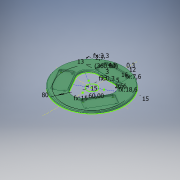
# Autodesk Inventor part: Stewart-Plate-inside
Saved by Autodesk Inventor 2018.2 (Build 222227000, 227)
## iProperties
Created: 2018-02-18
Part Number: Stewart-Plate-inside
Material: Generisch
Document SubType Name: Modeling
Designer: JochenAlt
Density: 1 g/cm^3
Appearance: Vorgabe
Author: JochenAlt
Autodesk Inventor part; units mm, degrees
ref_plane "YZ Plane" through (0, 0, 0) normal (1, 0, 0) x (0, 1, 0)
ref_plane "XZ Plane" through (0, 0, 0) normal (0, 1, 0) x (-1, 0, 0)
ref_plane "XY Plane" through (0, 0, 0) normal (0, 0, 1) x (1, 0, 0)
sketch "Skizze1" plane through (0, 0, 0) normal (0, 0, 1) x (1, 0, 0)
  line L0 (-56, 0) -> (56, 0) construction
  circle A0 centre (0, 0) radius 40
  line L1 (-8, 36) -> (8, 36)
  line L2 (8, 36) -> (8, 33)
  line L3 (8, 33) -> (-8, 33)
  line L4 (-8, 33) -> (-8, 36)
  line L5 (1.5, 33) -> (-1.5, 33)
  line L6 (-1.5, 33) -> (-1.5, 28)
  line L7 (-1.5, 28) -> (1.5, 28)
  line L8 (1.5, 28) -> (1.5, 33)
  circle A1 centre (0, 0) radius 7.5
  dimension "d9" = 80
  dimension "d10" = 3
  dimension "d11" = 33
  dimension "d14" = 16
  dimension "d23" = 5
  dimension "d62" = 15
  constraints: 16 end point, 4 parallel, 3 perpendicular, 2 centre point, 2 horizontal, 1 coincident, 1 midpoint, 1 point on line
  measures "d9" diameter of A0
  measures "d10" distance between parallel lines of L3 L1
  measures "d11" distance from line of L3 A0.centre
  measures "d14" distance between parallel lines of L2 L4
  measures "d23" distance between parallel lines of L3 L7
  measures "d62" diameter of A1
extrude "Extrusion3" add sketch "Skizze1" against normal blind 7 contours L1 L2 L3 L4 | L3 L8 L7 L6
fillet "Rundung1" radius 4 2 edges at (-8, 34.5, -7) (8, 34.5, -7)
sketch "Skizze2" plane through (-8, 36, 0) normal (0, 1, 0) x (1, 0, 0)
  circle A0 centre (3, 4) radius 1.1
  circle A1 centre (13, 4) radius 1.1
  line L0 (8, 0) -> (8, 7) construction
  line L1 (43, 0) -> (-27, 0) construction
  line L2 (-1.6221, 4) -> (19.0112, 4) construction
  line L3 (4, 7) -> (12, 7) construction
  line L4 (0, 0) -> (0, 3) projected
  dimension "d16" = 2.2
  dimension "d20" = 3
  dimension "d21" = 3
  constraints: 4 end point, 2 centre point, 1 equal radius, 1 horizontal, 1 midpoint, 1 point on line, 1 symmetric about line, 1 vertical
  measures "d16" diameter of A0
  measures "d20" distance between parallel lines of L3 L2
  measures "d21" distance from line of L4 A0.centre
extrude "Extrusion4" cut sketch "Skizze2" against normal up to next
chamfer "Fase1" distance 5 distance2 7 1 edges at (0, 28, -7) measured on face at (0, 28.5, -7)
pattern_circular "Runde Anordnung1" count 3 over 360 about axis through (0, 0, -10) along (0, 0, 1) of "Extrusion3", "Extrusion4", "Fase1", "Rundung1"
sketch "Skizze3" plane through (0, 0, 0) normal (0, 0, 1) x (1, 0, 0)
  line L0 (0, 70.94) -> (0, -77.1567) construction
  circle A0 centre (0, 0) radius 40 construction
  circle A1 centre (0, 0) radius 49.7834
  line L1 (12.1244, 22) -> (-12.1244, 22)
  line L2 (-25.1147, -0.5) -> (-12.9904, -21.5)
  line L3 (25.1147, -0.5) -> (12.9904, -21.5)
  line L4 (-25.1147, 14.5) -> (19.0526, -11) construction
  line L5 (38.1051, 22) -> (-19.0526, -11) construction
  arc A2 (25.1147, -0.5) -> (12.1244, 22) centre (12.1244, 7) ccw
  arc A3 (-12.1244, 22) -> (-25.1147, -0.5) centre (-12.1244, 7) ccw
  arc A4 (-12.9904, -21.5) -> (12.9904, -21.5) centre (0, -14) ccw
  line L6 (0.15, 50.4) -> (12.15, 50.4) construction
  line L7 (12.15, 50.4) -> (12.15, 23.8) construction
  line L8 (12.15, 23.8) -> (0.15, 23.8) construction
  line L9 (0.15, 23.8) -> (0.15, 50.4) construction
  line L10 (-0.15, 50.4) -> (-12.15, 50.4) construction
  line L11 (-12.15, 50.4) -> (-12.15, 23.8) construction
  line L12 (-12.15, 23.8) -> (-0.15, 23.8) construction
  line L13 (-0.15, 23.8) -> (-0.15, 50.4) construction
  line L14 (-17.45, 42.1) -> (17.45, 42.1)
  line L15 (19.75, 39.8) -> (19.75, 25.8)
  line L16 (17.45, 23.5) -> (-17.45, 23.5)
  line L17 (-19.75, 25.8) -> (-19.75, 39.8)
  arc A5 (-17.45, 42.1) -> (-19.75, 39.8) centre (-17.45, 39.8) ccw
  arc A6 (-19.75, 25.8) -> (-17.45, 23.5) centre (-17.45, 25.8) ccw
  arc A7 (17.45, 23.5) -> (19.75, 25.8) centre (17.45, 25.8) ccw
  arc A8 (19.75, 39.8) -> (17.45, 42.1) centre (17.45, 39.8) ccw
  circle A9 centre (-16.95, 39.45) radius 1.35
  circle A10 centre (-16.95, 26.45) radius 1.35
  circle A11 centre (16.95, 39.45) radius 1.35
  circle A12 centre (16.95, 26.45) radius 1.35
  line L18 (-19.75, 32.95) -> (19.75, 32.95) construction
  line L19 (-16.95, 39.45) -> (-16.95, 26.45) construction
  arc A13 (-27.7347, -36.1621) -> (-24.5928, -37.004) centre (-25.7428, -35.0121) ccw
  line L20 (-12.4685, -30.004) -> (-24.5928, -37.004)
  circle A14 centre (-25.6897, -34.4041) radius 1.35
  line L21 (-27.7347, -36.1621) -> (-45.1847, -5.9379)
  circle A15 centre (-14.4314, -27.9041) radius 1.35
  arc A16 (-12.4685, -30.004) -> (-11.6266, -26.8621) centre (-13.6185, -28.0121) ccw
  line L22 (-29.0766, 3.3621) -> (-11.6266, -26.8621)
  arc A17 (-29.0766, 3.3621) -> (-32.2185, 4.204) centre (-31.0685, 2.2121) ccw
  circle A18 centre (-31.3814, 1.4541) radius 1.35
  arc A19 (-44.3428, -2.796) -> (-45.1847, -5.9379) centre (-43.1928, -4.7879) ccw
  circle A20 centre (-42.6397, -5.0459) radius 1.35
  line L23 (-44.3428, -2.796) -> (-32.2185, 4.204)
  arc A21 (45.1847, -5.9379) -> (44.3428, -2.796) centre (43.1928, -4.7879) ccw
  line L24 (32.2185, 4.204) -> (44.3428, -2.796)
  circle A22 centre (42.6397, -5.0459) radius 1.35
  line L25 (45.1847, -5.9379) -> (27.7347, -36.1621)
  circle A23 centre (31.3814, 1.4541) radius 1.35
  arc A24 (32.2185, 4.204) -> (29.0766, 3.3621) centre (31.0685, 2.2121) ccw
  line L26 (11.6266, -26.8621) -> (29.0766, 3.3621)
  arc A25 (11.6266, -26.8621) -> (12.4685, -30.004) centre (13.6185, -28.0121) ccw
  circle A26 centre (14.4314, -27.9041) radius 1.35
  arc A27 (24.5928, -37.004) -> (27.7347, -36.1621) centre (25.7428, -35.0121) ccw
  circle A28 centre (25.6897, -34.4041) radius 1.35
  line L27 (24.5928, -37.004) -> (12.4685, -30.004)
  point P0 (-38.1051, 22)
  point P1 (0, -44)
  point P2 (-18.6605, -33.579)
  point P3 (-38.4105, 0.629)
  point P4 (38.4105, 0.629)
  point P5 (18.6605, -33.579)
  dimension "d140" = 60
  dimension "d141" = 15
  dimension "d144" = 15
  dimension "d146" = 0.3
  dimension "d147" = 26.6
  dimension "d148" = 12
  dimension "d150" = 0.3
  dimension "d151" = 18.6
  dimension "d152" = 2.3
  dimension "d153" = 13
  dimension "d154" = 7.6
  dimension "d155" = 4.8
  dimension "d158" = 360
  dimension "d160" = 1.5
  dimension "d161" = 2.7
  constraints: 54 end point, 31 point on circle, 28 centre point, 15 point on line, 14 tangent, 7 equal radius, 6 parallel, 4 perpendicular, 3 horizontal, 2 collinear, 2 midpoint, 2 symmetric about line, 1 coincident, 1 vertical, 97 other
  measures "d140" angle of L3 L1
  measures "d141" radius of A2
  measures "d144" radius of A4
  measures "d146" distance between parallel lines of L9 L13
  measures "d147" distance between parallel lines of L8 L6
  measures "d148" distance between parallel lines of L7 L9
  measures "d150" distance between parallel lines of L16 L8
  measures "d151" distance between parallel lines of L16 L14
  measures "d152" radius of A5
  measures "d153" distance of L19.end L19.start
  measures "d154" distance between parallel lines of L15 L7
  measures "d155" distance between parallel lines of L11 L19
  measures "d160" distance between parallel lines of L1 L16
  measures "d161" diameter of A9
extrude "Extrusion9" add sketch "Skizze3" along normal blind 4 contours A1
extrude "Extrusion6" add sketch "Skizze3" along normal blind 2 contours L14 A8 L15 A7 L16 A6 L17 A5 | L21 A19 L23 A17 L22 A16 L20 A13 | L25 A27 L27 A25 L26 A24 L24 A21
fillet "Rundung4" radius 1 14 edges at (19.0526, -11, 4) (0, -29, 4) (-19.0526, -11, 4) (-25.1147, 14.5, 4) (0, 22, 4) (25.1147, 14.5, 4) (-49.7834, 0, 4) (-49.7834, 0, 0) (25.1147, 14.5, 0) (0, 22, 0) (19.0526, -11, 0) (0, -29, 0) (-19.0526, -11, 0) (-25.1147, 14.5, 0)
equation "\"d21\" = d20"
